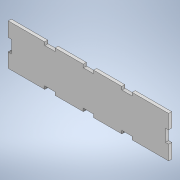
# Autodesk Inventor part: Стекнка t1
Saved by Autodesk Inventor 2021 (Build 250183000, 183)
## iProperties
Created: 2021-04-10
Part Number: Стекнка t1
Material: Типовые
Document SubType Name: Modeling
Designer: user
Density: 1 g/cm^3
Appearance: По умолчанию
Author: user
Autodesk Inventor part; units mm, degrees
ref_plane "YZ Plane" through (0, 0, 0) normal (1, 0, 0) x (0, 1, 0)
ref_plane "XZ Plane" through (0, 0, 0) normal (0, 1, 0) x (-1, 0, 0)
ref_plane "XY Plane" through (0, 0, 0) normal (0, 0, 1) x (1, 0, 0)
sketch "Эскиз1" plane through (0, 0, 0) normal (0, 0, 1) x (1, 0, 0)
  line L0 (-78.0042, 6) -> (-78.0042, 20)
  line L1 (-78.0042, 20) -> (-42.5, 20)
  line L2 (-32.5, 20) -> (-32.5, 17)
  line L3 (-32.5, 17) -> (-42.5, 17)
  line L4 (-42.5, 17) -> (-42.5, 20)
  line L5 (-32.5, 20) -> (-5, 20)
  line L6 (0, 17) -> (-5, 17)
  line L7 (-5, 17) -> (-5, 20)
  line L8 (-75.0118, -6.0217) -> (-75.0118, 6)
  line L9 (-75.0118, 6) -> (-78.0042, 6)
  line L10 (-78.0042, 20) -> (-42.5, 20)
  line L11 (-32.5, 20) -> (-5, 20)
  line L12 (77.9946, 6.1624) -> (77.9946, 20)
  line L13 (77.9946, 20) -> (42.5, 20)
  line L14 (32.5, 20) -> (32.5, 17)
  line L15 (32.5, 17) -> (42.5, 17)
  line L16 (42.5, 17) -> (42.5, 20)
  line L17 (32.5, 20) -> (5, 20)
  line L18 (0, 17) -> (5, 17)
  line L19 (5, 17) -> (5, 20)
  line L20 (74.9946, 0.1624) -> (74.9946, 6.1624)
  line L21 (74.9946, 6.1624) -> (77.9946, 6.1624)
  line L22 (77.9946, 20) -> (42.5, 20)
  line L23 (32.5, 20) -> (5, 20)
  line L24 (-78.0038, -6.0216) -> (-78.0038, -20)
  line L25 (-78.0038, -20) -> (-42.5, -20)
  line L26 (-32.5, -20) -> (-32.5, -17)
  line L27 (-32.5, -17) -> (-42.5, -17)
  line L28 (-42.5, -17) -> (-42.5, -20)
  line L29 (-32.5, -20) -> (-5, -20)
  line L30 (0, -17) -> (-5, -17)
  line L31 (-5, -17) -> (-5, -20)
  line L32 (-75.0118, -6.0217) -> (-75.0118, -6.0216)
  line L33 (-75.0118, -6.0216) -> (-78.0038, -6.0216)
  line L34 (-78.0038, -20) -> (-42.5, -20)
  line L35 (-32.5, -20) -> (-5, -20)
  line L36 (77.9946, -5.8376) -> (77.9946, -20)
  line L37 (77.9946, -20) -> (42.5, -20)
  line L38 (32.5, -20) -> (32.5, -17)
  line L39 (32.5, -17) -> (42.5, -17)
  line L40 (42.5, -17) -> (42.5, -20)
  line L41 (32.5, -20) -> (5, -20)
  line L42 (0, -17) -> (5, -17)
  line L43 (5, -17) -> (5, -20)
  line L44 (74.9946, 0.1624) -> (74.9946, -5.8376)
  line L45 (74.9946, -5.8376) -> (77.9946, -5.8376)
  line L46 (77.9946, -20) -> (42.5, -20)
  line L47 (32.5, -20) -> (5, -20)
  line L48 (-78.0042, 6) -> (-75.0042, 6)
  point P0 (0, 0)
  constraints: 98 end point, 2 horizontal, 1 parallel, 1 point on line
extrude "Выдавливание1" add sketch "Эскиз1" along normal blind 3
